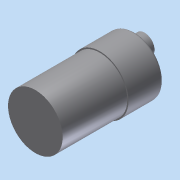
# Autodesk Inventor part: Motorbase
Saved by Autodesk Inventor 2012 (Build 160160000, 160)
## iProperties
Created: 2011-10-28
Part Number: Motorbase
Material: Default
Document SubType Name: Modeling
Designer: Kyle
Density: 1 g/cm^3
Author: Kyle
Autodesk Inventor part; units mm, degrees
ref_plane "YZ Plane" through (0, 0, 0) normal (1, 0, 0) x (0, 1, 0)
ref_plane "XZ Plane" through (0, 0, 0) normal (0, 1, 0) x (-1, 0, 0)
ref_plane "XY Plane" through (0, 0, 0) normal (0, 0, 1) x (1, 0, 0)
sketch "Sketch1" plane through (0, 0, 0) normal (0, 0, 1) x (1, 0, 0)
  circle A0 centre (0, 0) radius 18.2563
  dimension "d0" = 36.5125
  constraints: 1 centre point, 1 coincident
  measures "d0" diameter of A0
extrude "Extrusion1" add sketch "Sketch1" along normal blind 22.225
sketch "Sketch2" plane through (0, 0, 22.225) normal (0, 0, 1) x (1, 0, 0)
  circle A0 centre (0, 0) radius 18.2562 projected
  circle A1 centre (0, 0) radius 17.4625
  dimension "d3" = 34.925
  constraints: 1 centre point, 1 coincident
  measures "d3" diameter of A1
extrude "Extrusion2" add sketch "Sketch2" along normal blind 41.275 contours A1
fillet "Fillet1" radius 1.5875 1 edges at (-18.2563, 0, 0)
sketch "Sketch3" plane through (0, 0, 0) normal (0, 0, -1) x (-1, 0, 0)
  circle A0 centre (0, 0) radius 16.6687 projected
  circle A1 centre (0, 7.9375) radius 6.35
  dimension "d7" = 12.7
  dimension "d8" = 7.9375
  constraints: 1 centre point
  measures "d7" diameter of A1
  measures "d8" distance of A0.centre A1.centre
extrude "Extrusion3" add sketch "Sketch3" along normal blind 6.35 contours A1
sketch "Sketch4" plane through (0, 7.9375, -6.35) normal (0, 0, -1) x (-1, 0, 0)
  circle A0 centre (0, 0) radius 6.35 projected
  circle A1 centre (0, 0) radius 3.175
  point P0 (0, -7.9375)
  dimension "d11" = 6.35
  constraints: 1 centre point, 1 coincident
  measures "d11" diameter of A1
hole "Hole1" at (0, 7.9375, -6.35) direction (0, 0, 1) diameter 6.35 depth 6.35
body "Solid1"
